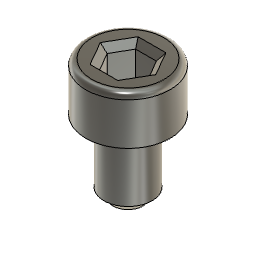
Spendenbox_Assebly v43 (Autodesk Fusion 360 archive; units mm, degrees)
design "DIN912_M4x06"
Autodesk Fusion 360 part; units mm, degrees
sketch "Sketch1" plane through (0, 0, 0) normal (0, 1, 0) x (1, 0, 0)
  line L0 (2, 0) -> (3.5, 0)
  line L1 (3.5, 0) -> (3.5, -4)
  line L2 (3.5, -4) -> (0, -4)
  line L3 (0, -4) -> (0, 6)
  line L4 (0, 6) -> (2, 6)
  line L5 (2, 6) -> (2, 0)
  dimension "d1" = 6
  dimension "d2" = 2
  dimension "d3" = 3.5
  dimension "d4" = 4
  constraint horizontal L0
  constraint perpendicular L0 L1
  constraint perpendicular L1 L2
  constraint perpendicular L2 L3
  constraint perpendicular L1 L4
  constraint vertical L5
  constraint coincident origin L0
  constraint coincident origin L3
  measures "d1" distance of L0.start L4.end
  measures "d2" distance of L3.end L4.end
  measures "d3" distance of L1.end L2.end
  measures "d4" distance of L0.end L1.end
revolve "Revolve1" add sketch "Sketch1" angle 360 about axis through (0, 0, 4) along (0, 0, -1)
sketch "Sketch3" plane through (0, 0, 4) normal (0, 0, 1) x (-1, 0, 0)
  circle A0 centre (0, 0) radius 3.5
  line L0 (-0.866, -1.5) -> (0.866, -1.5)
  line L1 (0.866, -1.5) -> (1.7321, 0)
  line L2 (1.7321, 0) -> (0.866, 1.5)
  line L3 (0.866, 1.5) -> (-0.866, 1.5)
  line L4 (-0.866, 1.5) -> (-1.7321, 0)
  line L5 (-1.7321, 0) -> (-0.866, -1.5)
  dimension "d6" = 3
  constraint coincident A0.centre origin
  constraint horizontal L0
  measures "d6" distance of L0 L3
extrude "Extrude1" cut sketch "Sketch3" against normal blind 4 contours L0 L1 L2 L3 L4 L5
chamfer "Chamfer1" distance 0.5 angle 45 6 edges at (1.299, -0.75, 4) (1.299, 0.75, 4) (0, 1.5, 4) (-1.299, 0.75, 4) (-1.299, -0.75, 4) (0, -1.5, 4)
fillet "Fillet1" radius 0.5 1 edges at (-3.2631, -1.2657, 4)
chamfer "Chamfer2" distance 0.75 angle 45 1 edges at (-1.8647, -0.7232, -6)
equation "d2 = ( 4 / 2 ) * 1 mm"
equation "d3 = ( 7 / 2 ) * 1 mm"

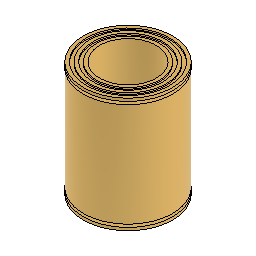
design "Brass_Insert_M4"
Autodesk Fusion 360 part; units mm, degrees
sketch "Skizze1" plane through (0, 0, 0) normal (0, 1, 0) x (1, 0, 0)
  line L0 (2, 0) -> (2, 8.1)
  line L1 (2, 0) -> (2.23, 0)
  line L2 (2.23, 0) -> (2.23, 0.1)
  line L3 (2.23, 0.1) -> (2.46, 0.1)
  line L4 (2.46, 0.1) -> (2.46, 0)
  line L5 (2.46, 0) -> (2.69, 0)
  line L6 (2.69, 0) -> (2.69, 0.1)
  line L7 (2.69, 0.1) -> (2.92, 0.1)
  line L8 (2.92, 0.1) -> (2.92, 0)
  line L9 (2.92, 0) -> (3.15, 0)
  line L10 (3.15, 0) -> (3.15, 0.2)
  line L11 (3.15, 0.2) -> (2.85, 0.2)
  line L12 (2.85, 0.2) -> (2.85, 0.4)
  line L13 (2.85, 0.4) -> (3.15, 0.4)
  line L14 (3.15, 0.4) -> (3.15, 7.7)
  line L15 (3.15, 7.7) -> (2.85, 7.7)
  line L16 (2.85, 7.7) -> (2.85, 7.9)
  line L17 (2.85, 7.9) -> (3.15, 7.9)
  line L18 (3.15, 7.9) -> (3.15, 8.1)
  line L19 (3.15, 8.1) -> (2, 8.1)
  line L20 (2, 4.05) -> (3.15, 4.05) construction
  dimension "d3" = 0.1
  dimension "d4" = 0.2
  dimension "d5" = 8.1
  dimension "d10" = 0.3
  dimension "d11" = 3.15
  dimension "d12" = 2
  constraint vertical L0
  constraint perpendicular L0 L1
  constraint perpendicular L1 L2
  constraint perpendicular L2 L3
  constraint perpendicular L3 L4
  constraint perpendicular L4 L5
  constraint perpendicular L3 L6
  constraint perpendicular L4 L7
  constraint perpendicular L7 L8
  constraint equal L5 L9
  constraint equal L1 L5
  constraint coincident origin L1
  constraint collinear L5 L9
  constraint collinear L1 L9
  constraint equal L3 L7
  constraint equal L5 L7
  constraint equal L4 L6
  constraint perpendicular L9 L10
  constraint perpendicular L10 L11
  constraint perpendicular L11 L12
  constraint perpendicular L12 L13
  constraint perpendicular L13 L14
  constraint perpendicular L14 L15
  constraint perpendicular L13 L16
  constraint perpendicular L14 L17
  constraint perpendicular L13 L18
  constraint horizontal L19
  constraint midpoint L0 L20.start
  constraint midpoint L14 L20.end
  constraint horizontal L20
  constraint equal L12 L16
  constraint equal L10 L12
  constraint collinear L10 L14
  constraint collinear L12 L16
  constraint collinear L10 L18
  measures "d3" distance of L5.end L6.end
  measures "d4" distance of L9.end L10.end
  measures "d5" distance of L9.end L18.end
  measures "d10" distance of L10.end L11.end
  measures "d11" distance of origin L9.end
  measures "d12" distance of origin L0.start
revolve "Drehen1" add sketch "Skizze1" angle 360 about axis through (0, 0, 1.75) along (0, 0, 1)
equation "d11 = ( 6.3 / 2 ) * 1 mm"
